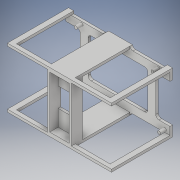
# Autodesk Inventor part: Rear Containment Thingy
Saved by Autodesk Inventor 2018.2 (Build 222227000, 227)
## iProperties
Created: 2018-04-10
Part Number: Rear Containment Thingy
Material: Generic
Document SubType Name: Modeling
Designer: MIABo
Density: 1 g/cm^3
Appearance: Default
Author: MIABo
Autodesk Inventor part; units mm, degrees
ref_plane "YZ Plane" through (0, 0, 0) normal (1, 0, 0) x (0, 1, 0)
ref_plane "XZ Plane" through (0, 0, 0) normal (0, 1, 0) x (-1, 0, 0)
ref_plane "XY Plane" through (0, 0, 0) normal (0, 0, 1) x (1, 0, 0)
sketch "Sketch1" plane through (0, 0, 0) normal (0, 0, 1) x (1, 0, 0)
  line L0 (50.8, 7.62) -> (50.8, 0)
  line L1 (50.8, 0) -> (-50.8, 0)
  line L2 (-50.8, 0) -> (-50.8, 7.62)
  line L3 (-29.21, 7.62) -> (-29.21, 45.72)
  line L4 (-36.83, 45.72) -> (-36.83, 7.62)
  line L5 (50.8, 45.72) -> (50.8, 53.34)
  line L6 (50.8, 53.34) -> (-50.8, 53.34)
  line L7 (-50.8, 53.34) -> (-50.8, 45.72)
  line L8 (29.21, 45.72) -> (29.21, 7.62)
  line L9 (36.83, 7.62) -> (36.83, 45.72)
  line L10 (-50.8, 45.72) -> (-36.83, 45.72)
  line L11 (-29.21, 45.72) -> (29.21, 45.72)
  line L12 (36.83, 45.72) -> (50.8, 45.72)
  line L13 (-50.8, 7.62) -> (-36.83, 7.62)
  line L14 (-29.21, 7.62) -> (29.21, 7.62)
  line L15 (36.83, 7.62) -> (50.8, 7.62)
  point P0 (0, 0)
  point P1 (0, 0)
  dimension "d2" = 101.6
  dimension "d3" = 7.62
  dimension "d6" = 13.97
  dimension "d7" = 7.62
  dimension "d8" = 7.62
  dimension "d9" = 13.97
  dimension "d10" = 7.62
  dimension "d12" = 38.1
  dimension "d13" = 0
  dimension "d14" = 38.1
  dimension "d15" = 0
  dimension "d16" = 38.1
  constraints: 32 end point, 10 parallel, 6 horizontal, 6 perpendicular, 2 collinear, 1 coincident, 1 midpoint
  measures "d2" distance of L0.end L1.end
  measures "d3" distance of L0.start L0.end
  measures "d6" distance between parallel lines of L2 L4
  measures "d7" distance of L5.end L5.start
  measures "d8" distance between parallel lines of L9 L8
  measures "d9" distance between parallel lines of L0 L9
  measures "d10" distance between parallel lines of L3 L4
  measures "d12" distance between parallel lines of L12 L15
  measures "d13" distance between parallel lines of L12 L11
  measures "d14" distance between parallel lines of L12 L14
  measures "d15" distance between parallel lines of L12 L10
  measures "d16" distance between parallel lines of L12 L13
extrude "Extrusion1" add sketch "Sketch1" along normal blind 2.54
sketch "Sketch2" plane through (0, 0, 2.54) normal (0, 0, 1) x (1, 0, 0)
  circle A0 centre (-36.83, 2.54) radius 1.524
  circle A1 centre (45.72, 2.54) radius 1.524
  circle A2 centre (-35.56, 50.8) radius 1.524
  circle A3 centre (39.37, 50.8) radius 1.524
  line L0 (-50.8, 0) -> (50.8, 0) projected
  line L1 (-50.8, 7.62) -> (-50.8, 0) projected
  line L2 (-50.8, 53.34) -> (-50.8, 45.72) projected
  line L3 (50.8, 53.34) -> (-50.8, 53.34) projected
  point P0 (0, 0)
  dimension "d19" = 3.048
  dimension "d21" = 2.54
  dimension "d22" = 2.54
  dimension "d25" = 13.97
  dimension "d26" = 96.52
  dimension "d27" = 15.24
  dimension "d28" = 2.54
  dimension "d29" = 90.17
  dimension "d30" = 2.54
  constraints: 4 centre point, 3 equal radius
  measures "d19" diameter of A0
  measures "d21" distance from line of L0 A0.centre
  measures "d22" distance from line of L0 A1.centre
  measures "d25" distance from line of L1 A0.centre
  measures "d26" distance from line of A1.centre L1
  measures "d27" distance from line of L2 A2.centre
  measures "d28" distance from line of L3 A2.centre
  measures "d29" distance from line of A3.centre L2
  measures "d30" distance from line of L3 A3.centre
extrude "Extrusion2" add sketch "Sketch2" along normal blind 5.588
sketch "Sketch3" plane through (0, 0, 0) normal (0, 0, -1) x (-1, 0, 0)
  line L0 (50.8, 0) -> (-50.8, 0) projected
  line L1 (11.6205, 0) -> (-11.6205, 0)
  line L2 (-11.6205, 0) -> (-11.6205, -2.54)
  line L3 (-11.6205, -2.54) -> (11.6205, -2.54)
  line L4 (11.6205, -2.54) -> (11.6205, 0)
  line L5 (-50.8, 53.34) -> (50.8, 53.34) projected
  line L6 (11.6205, 53.34) -> (-11.6205, 53.34)
  line L7 (-11.6205, 53.34) -> (-11.6205, 55.88)
  line L8 (-11.6205, 55.88) -> (11.6205, 55.88)
  line L9 (11.6205, 55.88) -> (11.6205, 53.34)
  line L10 (-50.8, 0) -> (-50.8, 7.62) projected
  line L11 (-50.8, 0) -> (-45.72, 0)
  line L12 (-45.72, 0) -> (-45.72, -2.54)
  line L13 (-45.72, -2.54) -> (-50.8, -2.54)
  line L14 (-50.8, -2.54) -> (-50.8, 0)
  line L15 (-50.8, 45.72) -> (-50.8, 53.34) projected
  line L16 (-50.8, 55.88) -> (-50.8, 55.88)
  line L17 (-50.8, 53.34) -> (-48.26, 53.34)
  line L18 (-50.8, 53.34) -> (-45.72, 53.34)
  line L19 (-45.72, 53.34) -> (-45.72, 55.88)
  line L20 (-45.72, 55.88) -> (-50.8, 55.88)
  line L21 (-50.8, 55.88) -> (-50.8, 53.34)
  line L22 (50.8, 7.62) -> (50.8, 0) projected
  line L23 (50.8, 0) -> (45.72, 0)
  line L24 (45.72, 0) -> (45.72, -2.54)
  line L25 (45.72, -2.54) -> (50.8, -2.54)
  line L26 (50.8, -2.54) -> (50.8, 0)
  line L27 (50.8, 53.34) -> (50.8, 45.72) projected
  line L28 (50.8, 53.34) -> (45.72, 53.34)
  line L29 (45.72, 53.34) -> (45.72, 55.88)
  line L30 (45.72, 55.88) -> (50.8, 55.88)
  line L31 (50.8, 55.88) -> (50.8, 53.34)
  point P0 (0, 0)
  point P1 (0, 0)
  dimension "d33" = 23.241
  dimension "d34" = 2.54
  dimension "d35" = 23.241
  dimension "d36" = 2.54
  dimension "d53" = 5.08
  dimension "d54" = 2.54
  dimension "d62" = 5.08
  dimension "d63" = 5.08
  dimension "d64" = 2.54
  dimension "d65" = 5.08
  constraints: 52 end point, 12 parallel, 7 horizontal, 6 perpendicular, 2 collinear, 2 midpoint, 2 point on line
  measures "d33" distance of L3.end L2.end
  measures "d34" distance of L3.end L1.start
  measures "d35" distance of L7.end L8.end
  measures "d36" distance of L6.end L7.end
  measures "d53" distance of L12.end L13.end
  measures "d54" distance of L11.end L12.end
  measures "d62" distance of L20.end L19.end
  measures "d63" distance of L25.end L24.end
  measures "d64" distance of L24.end L23.end
  measures "d65" distance of L29.end L30.end
extrude "Extrusion3" add sketch "Sketch3" against normal blind 59.69
fillet "Fillet1" radius 3.175 12 edges at (-11.6205, 0, 1.27) (11.6205, 0, 1.27) (11.6205, 53.34, 1.27) (-11.6205, 53.34, 1.27) (29.21, 45.72, 1.27) (36.83, 45.72, 1.27) (36.83, 7.62, 1.27) (29.21, 7.62, 1.27) (-29.21, 7.62, 1.27) (-29.21, 45.72, 1.27) (-36.83, 45.72, 1.27) (-36.83, 7.62, 1.27)
sketch "Sketch4" plane through (0, 0, 59.69) normal (0, 0, 1) x (1, 0, 0)
  line L0 (-11.6205, 0) -> (11.6205, 0) projected
  line L1 (11.6205, 53.34) -> (-11.6205, 53.34) projected
  line L2 (-11.6205, 0) -> (11.6205, 0)
  line L3 (11.6205, 0) -> (11.6205, 53.34)
  line L4 (11.6205, 53.34) -> (-11.6205, 53.34)
  line L5 (-11.6205, 53.34) -> (-11.6205, 0)
  line L6 (-9.525, 1.27) -> (9.525, 1.27)
  line L7 (9.525, 1.27) -> (9.525, 52.07)
  line L8 (9.525, 52.07) -> (-9.525, 52.07)
  line L9 (-9.525, 52.07) -> (-9.525, 1.27)
  point P0 (0, 0)
  dimension "d40" = 19.05
  dimension "d41" = 50.8
  dimension "d42" = 1.27
  dimension "d43" = 2.0955
  constraints: 16 end point, 4 parallel, 2 horizontal, 2 perpendicular
  measures "d40" distance of L8.end L7.end
  measures "d41" distance of L7.end L6.end
  measures "d42" distance between parallel lines of L6 L0
  measures "d43" distance between parallel lines of L5 L9
extrude "Extrusion4" add sketch "Sketch4" against normal blind 8.255
sketch "Sketch5" plane through (0, 0, 51.435) normal (0, 0, -1) x (-1, 0, 0)
  line L0 (11.6205, 0) -> (11.6205, 53.34) projected
  line L1 (-11.6205, 0) -> (11.6205, 0)
  line L2 (11.6205, 0) -> (11.6205, 53.34)
  line L3 (11.6205, 53.34) -> (-11.6205, 53.34)
  line L4 (-11.6205, 53.34) -> (-11.6205, 0)
  point P0 (0, 0)
  constraints: 8 end point, 2 parallel, 1 horizontal, 1 perpendicular
extrude "Extrusion5" add sketch "Sketch5" along normal blind 2.54
sketch "Sketch6" plane through (0, 0, 51.435) normal (0, 0, 1) x (1, 0, 0)
  line L0 (-9.525, 17.145) -> (9.525, 17.145)
  line L1 (9.525, 17.145) -> (9.525, 36.195)
  line L2 (9.525, 36.195) -> (-9.525, 36.195)
  line L3 (-9.525, 36.195) -> (-9.525, 17.145)
  line L4 (-9.525, 1.27) -> (-9.525, 52.07) projected
  line L5 (9.525, 1.27) -> (-9.525, 1.27) projected
  point P0 (0, 0)
  dimension "d48" = 19.05
  dimension "d49" = 19.05
  dimension "d50" = 15.875
  constraints: 8 end point, 2 parallel, 1 collinear, 1 horizontal, 1 perpendicular
  measures "d48" distance of L2.end L1.end
  measures "d49" distance of L1.end L0.end
  measures "d50" distance between parallel lines of L5 L0
extrude "Extrusion6" cut sketch "Sketch6" against normal blind 2.794
sketch "Sketch7" plane through (45.72, -2.54, 0) normal (-1, 0, 0) x (0, 0, 1)
  line L0 (2.54, 2.54) -> (59.69, 2.54) projected
  line L1 (59.69, 2.54) -> (55.88, 2.54)
  line L2 (55.88, 2.54) -> (55.88, 0)
  line L3 (55.88, 0) -> (59.69, 0)
  line L4 (59.69, 0) -> (59.69, 2.54)
  line L5 (0, 58.42) -> (59.69, 58.42) projected
  line L6 (2.54, 55.88) -> (59.69, 55.88) projected
  line L7 (59.69, 58.42) -> (55.88, 58.42)
  line L8 (55.88, 58.42) -> (55.88, 55.88)
  line L9 (55.88, 55.88) -> (59.69, 55.88)
  line L10 (59.69, 55.88) -> (59.69, 58.42)
  point P0 (0, 2.54)
  dimension "d66" = 3.81
  dimension "d67" = 2.54
  dimension "d68" = 3.81
  constraints: 16 end point, 4 parallel, 2 horizontal, 2 perpendicular, 1 point on line
  measures "d66" distance of L3.end L2.end
  measures "d67" distance of L2.end L1.end
  measures "d68" distance of L9.end L8.end
extrude "Extrusion7" add sketch "Sketch7" along normal up to surface (91.44 mm away)
body "Solid1"
